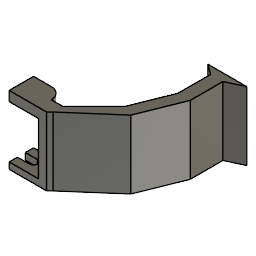
leg sprint 5 (Autodesk Fusion 360 design; units mm, degrees)
Autodesk Fusion 360 part; units mm, degrees
note: some values were not read from the file. Chosen so that the rebuilt part matches the saved one: which face or edge a step refers to; which pieces of a blend or face edit are solid.
sketch "Sketch1" plane through (0, 0, 0) normal (0, 0, 1) x (1, 0, 0)
  line L0 (0, 0) -> (50, 0)
  line L1 (50, 0) -> (50, 15)
  line L2 (50, 15) -> (0, 15)
  line L3 (0, 15) -> (0, 0)
  constraint horizontal L0
  constraint vertical L1
  constraint horizontal L2
  constraint vertical L3
  constraint coincident L0.start L3.end
extrude "Extrude1" add sketch "Sketch1" along normal blind 40 contours L0 L1 L2 L3 picked at (16.666667, 5)
sketch "Sketch2" plane through (0, 0, 0) normal (-1, 0, 0) x (0, -1, 0)
  line L0 (-15, 0) -> (0, 0)
  line L1 (0, 0) -> (0, 40)
  line L2 (0, 40) -> (-15, 40)
  line L3 (-15, 40) -> (-15, 0)
  line L4 (2.957876, 2) -> (-22.207484, 2)
  line L5 (-22.207484, 2) -> (-22.207484, 38.000001)
  line L6 (-22.207484, 38.000001) -> (2.957876, 38.000001)
  line L7 (2.957876, 38.000001) -> (2.957876, 2)
  constraint horizontal L4
  constraint vertical L5
  constraint horizontal L6
  constraint vertical L7
extrude "Extrude2" cut sketch "Sketch2" against normal blind 46 contours L1 L3 L4 L6 picked at (-10, 26)
sketch "Sketch3" plane through (0, 0, 40) normal (0, 0, 1) x (-1, 0, 0)
  line L0 (0, -15) -> (0, 0)
  line L1 (0, 0) -> (-50, 0)
  line L2 (-50, 0) -> (-50, -15)
  line L3 (-50, -15) -> (0, -15)
  circle A0 centre (-7.5, -7.5) radius 2.4
  dimension "d5" = 4.8
  measures "d5" diameter of A0
extrude "Extrude3" cut sketch "Sketch3" against normal blind 50 contours A0 picked at (-7.452057, -6.860244)
sketch "Sketch4" plane through (0, 0, 0) normal (0, 0, -1) x (1, 0, 0)
  circle A0 centre (7.5, -7.5) radius 2.4
  line L0 (0, 0) -> (0, -15)
  line L1 (0, -15) -> (50, -15)
  line L2 (50, -15) -> (50, 0)
  line L3 (50, 0) -> (0, 0)
  circle A1 centre (7.5, -7.5) radius 4
  dimension "d8" = 8
  constraint concentric A0 A1
  measures "d8" diameter of A1
extrude "Extrude4" cut sketch "Sketch4" against normal blind 7 contours A1 picked at (10.951775, -7.698723)
extrude "Extrude5" add 1 faces at (46, 10, 26) along direction (-1, 0, 0) blind 30
extrude "Extrude6" cut 1 faces at (50, 5, 26.666667) along direction (-1, 0, 0) blind 25
chamfer "Chamfer1" distance 7 angle 45 1 edges at (25, 15, 20)
chamfer "Chamfer2" distance 2 angle 45 1 edges at (25, 0, 20)
extrude "Extrude7" add 1 faces at (22.666667, 10.333333, 13.333333) along direction (0.70710678, 0.70710678, 0) blind 30
chamfer "Chamfer3" distance 7 angle 45 1 edges at (39.213203, 36.213203, 20)
extrude "Extrude8" add 1 faces at (40.863119, 31.263456, 13.333333) along direction (0, 1, 0) blind 25
sketch "Sketch5" plane through (0, 0, 0) normal (0, 0, -1) x (1, 0, 0)
  circle A0 centre (7.5, -7.5) radius 4
  line L0 (44.162951, -31.263456) -> (46.213203, -29.213203)
  line L1 (46.213203, -29.213203) -> (25, -8)
  line L2 (25, -8) -> (25, -2)
  line L3 (25, -2) -> (23, 0)
  line L4 (23, 0) -> (0, 0)
  line L5 (0, 0) -> (0, -15)
  line L6 (0, -15) -> (18, -15)
  line L7 (18, -15) -> (34.263456, -31.263456)
  line L8 (34.263456, -31.263456) -> (34.263456, -56.263456)
  line L9 (34.263456, -56.263456) -> (44.162951, -56.263456)
  line L10 (44.162951, -56.263456) -> (44.162951, -31.263456)
  line L11 (44.162951, -31.263456) -> (44.162951, -27.162951)
  line L12 (44.162951, -27.162951) -> (46.213203, -29.213203)
  line L13 (44.162951, -31.263456) -> (46.213203, -29.213203)
  constraint parallel L10 L11
extrude "Extrude9" cut sketch "Sketch5" against normal blind 43 contours L0 L1 L11 L12 L13 picked at (44.846368, -29.213203)
chamfer "Chamfer4" distance 3 angle 45 1 edges at (44.162951, 56.263456, 20)
sketch "Sketch6" plane through (0, 0, 0) normal (0, 0, -1) x (1, 0, 0)
  line L0 (41.162951, -56.263456) -> (44.162951, -53.263456)
  line L1 (44.162951, -53.263456) -> (44.162951, -27.162951)
  line L2 (44.162951, -27.162951) -> (25, -8)
  line L3 (25, -8) -> (25, -2)
  line L4 (25, -2) -> (23, 0)
  line L5 (23, 0) -> (0, 0)
  line L6 (0, 0) -> (0, -15)
  line L7 (0, -15) -> (18, -15)
  line L8 (18, -15) -> (34.263456, -31.263456)
  line L9 (34.263456, -31.263456) -> (34.263456, -56.263456)
  line L10 (34.263456, -56.263456) -> (41.162951, -56.263456)
  circle A0 centre (7.5, -7.5) radius 4
  circle A1 centre (7.5, -7.5) radius 2.4
  dimension "d25" = 4.8
  constraint concentric A0 A1
  measures "d25" diameter of A1
extrude "Extrude10" add sketch "Sketch6" against normal blind 2 contours A0 picked at (10.951775, -7.698723)
sketch "Sketch7" plane through (0, 0, 38.000001) normal (0, 0, -1) x (1, 0, 0)
  line L0 (16, -15) -> (16, 0)
  line L1 (16, 0) -> (0, 0)
  line L2 (0, 0) -> (0, -15)
  line L3 (0, -15) -> (16, -15)
  circle A0 centre (7.5, -7.5) radius 2.4
  circle A1 centre (7.5, -7.5) radius 4
  dimension "d28" = 8
  constraint concentric A0 A1
  measures "d28" diameter of A1
extrude "Extrude11" cut sketch "Sketch7" against normal blind 3 contours A1 picked at (10.951775, -7.698723)
sketch "Sketch8" plane through (0, 0, 38.000001) normal (0, 0, -1) x (1, 0, 0)
  circle A0 centre (7.5, -7.5) radius 4
  line L0 (16, -15) -> (16, 0)
  line L1 (16, 0) -> (0, 0)
  line L2 (0, 0) -> (0, -15)
  line L3 (0, -15) -> (16, -15)
  circle A1 centre (7.5, -7.5) radius 4
  constraint concentric A0 A1
extrude "Extrude12" add sketch "Sketch8" along normal blind 2 and the other way blind 2 contours A0 A1 picked at (6.101654, -8.048811)
extrude "Extrude13" cut 1 faces at (36.563288, 56.263456, 26.666667) along direction (0, -1, 0) blind 25
sketch "Sketch9" plane through (0, 0, 40) normal (0, 0, 1) x (-1, 0, 0)
  line L0 (-41.162951, -56.263456) -> (-41.162951, -31.263456)
  line L1 (-41.162951, -31.263456) -> (-34.263456, -31.263456)
  line L2 (-34.263456, -31.263456) -> (-18, -15)
  line L3 (-18, -15) -> (0, -15)
  line L4 (0, -15) -> (0, 0)
  line L5 (0, 0) -> (-23, 0)
  line L6 (-23, 0) -> (-25, -2)
  line L7 (-25, -2) -> (-25, -8)
  line L8 (-25, -8) -> (-44.162951, -27.162951)
  line L9 (-44.162951, -27.162951) -> (-44.162951, -53.263456)
  line L10 (-44.162951, -53.263456) -> (-41.162951, -56.263456)
extrude "Extrude14" cut 1 faces at (41.162951, 47.930123, 13.333333) along direction (1, 0, 0) blind 26
sketch "Sketch10" plane through (0, 0, 40) normal (0, 0, 1) x (-1, 0, 0)
  line L0 (-44.000001, -27) -> (-34.000001, -31)
  line L1 (-34.000001, -31) -> (-34.243008, -31.24155)
  line L2 (-34.243008, -31.24155) -> (-44.199999, -31.24155)
  line L3 (-44.199999, -31.24155) -> (-44.199999, -27.099999)
  line L4 (-44.199999, -27.099999) -> (-44.000001, -27)
  constraint horizontal L2
  constraint perpendicular L2 L3
extrude "Extrude15" cut sketch "Sketch10" against normal blind 45 contours L0 L1 L2 L3 L4 picked at (-40.814336, -29.8277)
delete_face "DeleteFace1" 1 faces at (40.863119, 31.263456, 13.333333)
delete_face "DeleteFace2" 1 faces at (40.856303, 34.548684, 40)
extrude "Extrude16" add 2 faces at (40.666667, 28.333334, 36.161338) (40.666667, 28.333334, 18.989342) along direction (0.37139068, 0.92847669, 0) blind 40
chamfer "Chamfer5" distance 5 angle 45 1 edges at (58.855628, 64.139068, 20)
extrude "Extrude17" add 1 faces at (13.966667, 7.5, 2) along direction (0, 0, 1) blind 4
extrude "Extrude18" cut 1 faces at (46.618101, 52.878584, 0) along direction (0, 0, 1) blind 2
extrude "Extrude19" cut 1 faces at (16, 10, 16.666667) along direction (1, 0, 0) blind 2
sketch "Sketch11" plane through (0, 0, 40) normal (0, 0, 1) x (-1, 0, 0)
  line L0 (-56.998674, -59.496685) -> (-54.213244, -65.996021)
  line L1 (-54.213244, -65.996021) -> (-48.855628, -68.139068)
  line L2 (-48.855628, -68.139068) -> (-34.000001, -31)
  line L3 (-34.000001, -31) -> (-18, -15)
  line L4 (-18, -15) -> (0, -15)
  line L5 (0, -15) -> (0, 0)
  line L6 (0, 0) -> (-23, 0)
  line L7 (-23, 0) -> (-25, -2)
  line L8 (-25, -2) -> (-25, -8)
  line L9 (-25, -8) -> (-44.000001, -27)
  line L10 (-44.000001, -27) -> (-56.998674, -59.496685)
  line L11 (-56.998674, -59.496685) -> (-60.937867, -50.305234)
  line L12 (-60.937867, -50.305234) -> (-50.499337, -24.208909)
  line L13 (-50.499337, -24.208909) -> (-25, -2)
  line L14 (-18, -15) -> (-18, -8)
  line L15 (-18, -8) -> (-25, -8)
  dimension "d50" = 10
  constraint parallel L0 L11
  constraint parallel L10 L12
  constraint coincident L7.end L8.start
  constraint coincident L3.end L4.start
  constraint perpendicular L4 L14
  constraint coincident L8.end L9.start
extrude "Extrude20" add sketch "Sketch11" against normal blind 38 contours L8 L9 L10 L11 L12 L13 picked at (-53.978847, -45.60064)
extrude "Extrude21" cut sketch "Sketch11" against normal blind 40 contours L0 L1 L2 L3 L9 L10 L14 L15 picked at (-46.618101, -52.878584)
extrude "Extrude22" add sketch "Sketch11" along normal blind 2 contours L8 L9 L10 L11 L12 L13 | L4 L5 L6 L7 L8 L14 L15 picked at (-53.978847, -45.60064) picked at (-6, -7.666667)
fillet "Fillet1" radius 7 2 edges at (18, 15, 4) (18, 15, 40)
sketch "Sketch15" plane through (0, 0, 42) normal (0, 0, 1) x (-1, 0, 0)
  arc A0 (-18, -8) -> (-11, -15) centre (-11, -8) ccw
  line L0 (-11, -15) -> (0, -15)
  line L1 (0, -15) -> (0, 0)
  line L2 (0, 0) -> (-23, 0)
  line L3 (-23, 0) -> (-25, -2)
  line L4 (-25, -2) -> (-50.499337, -24.208909)
  line L5 (-50.499337, -24.208909) -> (-60.937867, -50.305234)
  line L6 (-60.937867, -50.305234) -> (-56.998674, -59.496685)
  line L7 (-56.998674, -59.496685) -> (-44.000001, -27)
  line L8 (-44.000001, -27) -> (-25, -8)
  line L9 (-25, -8) -> (-18, -8)
  line L10 (-60.937867, -50.305234) -> (-53.322094, -50.305234)
  line L11 (-53.322094, -50.305234) -> (-56.998674, -59.496685)
  line L12 (-61.161175, -50.305234) -> (-56.998674, -59.496685)
  line L13 (-61.161175, -50.305234) -> (-60.899999, -50.305234)
  constraint horizontal L10
  constraint parallel L10 L13
extrude "Extrude23" cut sketch "Sketch15" against normal blind 41 contours L6 L7 L10 L11 L13 picked at (-57.073589, -53.369051)
extrude "Extrude24" add 1 faces at (58.399276, 50.305234, 28.666667) along direction (0, 1, 0) blind 20
sketch "Sketch16" plane through (0, 0, 2) normal (0, 0, -1) x (1, 0, 0)
  circle A0 centre (7.5, -7.5) radius 2.4
  line L0 (60.937867, -50.305234) -> (50.499337, -24.208909)
  line L1 (50.499337, -24.208909) -> (25, -2)
  line L2 (25, -2) -> (23, 0)
  line L3 (23, 0) -> (0, 0)
  line L4 (0, 0) -> (0, -15)
  line L5 (0, -15) -> (11, -15)
  arc A1 (11, -15) -> (18, -8) centre (11, -8) ccw
  line L6 (18, -8) -> (25, -8)
  line L7 (25, -8) -> (44.000001, -27)
  line L8 (44.000001, -27) -> (53.322094, -50.305234)
  line L9 (53.322094, -50.305234) -> (53.322094, -70.305234)
  line L10 (53.322094, -70.305234) -> (60.937867, -70.305234)
  line L11 (60.937867, -70.305234) -> (60.937867, -50.305234)
  line L12 (71.000001, -75.000001) -> (60.937867, -70.305234)
  line L13 (53.322094, -70.305234) -> (47.000001, -75.000001)
  line L14 (47.000001, -75.000001) -> (71.000001, -75.000001)
  constraint perpendicular L9 L14
extrude "Extrude25" add sketch "Sketch16" against normal blind 40 contours L10 L12 L13 L14 picked at (59.645956, -73.435079)
extrude "Extrude31" cut 1 faces at (6.101654, 8.048811, 36.000001) along direction (0, 0, 1) blind 1
sketch "Sketch17" plane through (0, 0, 2) normal (0, 0, -1) x (1, 0, 0)
  circle A0 centre (7.5, -7.5) radius 2.4
  line L0 (60.937867, -50.305234) -> (50.499337, -24.208909)
  line L1 (50.499337, -24.208909) -> (25, -2)
  line L2 (25, -2) -> (23, 0)
  line L3 (23, 0) -> (0, 0)
  line L4 (0, 0) -> (0, -15)
  line L5 (0, -15) -> (11, -15)
  arc A1 (11, -15) -> (18, -8) centre (11, -8) ccw
  line L6 (18, -8) -> (25, -8)
  line L7 (25, -8) -> (44.000001, -27)
  line L8 (44.000001, -27) -> (53.322094, -50.305234)
  line L9 (53.322094, -50.305234) -> (53.322094, -70.305234)
  line L10 (53.322094, -70.305234) -> (47.000001, -75.000001)
  line L11 (47.000001, -75.000001) -> (71.000001, -75.000001)
  line L12 (71.000001, -75.000001) -> (60.937867, -70.305234)
  line L13 (60.937867, -70.305234) -> (60.937867, -50.305234)
  line L14 (7.5, -5.1) -> (0, -5.1)
  line L15 (7.5, -9.9) -> (0, -9.9)
  line L16 (0, -9.9) -> (0, -5.1)
  constraint coincident A0 L14.start
  constraint coincident L4 L14.end
  constraint perpendicular L4 L14
  constraint coincident A0 L15.start
  constraint coincident L4 L15.end
  constraint perpendicular L4 L15
extrude "Extrude32" cut sketch "Sketch17" against normal blind 4 contours A0 L4 L14 L15 L16 picked at (1.702237, -7.440216)
sketch "Sketch18" plane through (0, 0, 37.000001) normal (0, 0, -1) x (1, 0, 0)
  circle A0 centre (7.5, -7.5) radius 4
  line L0 (8.5, -7.5) -> (8.5, -3.627017)
  line L1 (8.5, -7.5) -> (8.5, -11.372983)
  line L2 (6.5, -7.5) -> (6.5, -3.627017)
  line L3 (6.5, -7.5) -> (6.5, -11.372983)
  constraint vertical L2
  constraint parallel L2 L3
extrude "Extrude33" cut sketch "Sketch18" against normal blind 1 contours A0 L0 L1 | A0 L2 L3 picked at (10.485726, -7.694579) picked at (4.514274, -7.305421)
fillet "Fillet2" radius 1 4 edges at (8.5, 3.627017, 37.500001) (8.5, 11.372983, 37.500001) (6.5, 3.627017, 37.500001) (6.5, 11.372983, 37.500001)
extrude "Extrude34" add 1 faces at (9.667133, 7.666667, 42) along direction (0, 0, 1) blind 2
sketch "Sketch19" plane through (0, 0, 44) normal (0, 0, 1) x (-1, 0, 0)
  line L0 (-53.322094, -50.305234) -> (-44.000001, -27)
  line L1 (-44.000001, -27) -> (-25, -8)
  line L2 (-25, -8) -> (-18, -8)
  arc A0 (-18, -8) -> (-11, -15) centre (-11, -8) ccw
  line L3 (-11, -15) -> (0, -15)
  line L4 (0, -15) -> (0, 0)
  line L5 (0, 0) -> (-23, 0)
  line L6 (-23, 0) -> (-25, -2)
  line L7 (-25, -2) -> (-50.499337, -24.208909)
  line L8 (-50.499337, -24.208909) -> (-60.937867, -50.305234)
  line L9 (-60.937867, -50.305234) -> (-60.937867, -70.305234)
  line L10 (-60.937867, -70.305234) -> (-71.000001, -75.000001)
  line L11 (-71.000001, -75.000001) -> (-47.000001, -75.000001)
  line L12 (-47.000001, -75.000001) -> (-53.322094, -70.305234)
  line L13 (-53.322094, -70.305234) -> (-53.322094, -50.305234)
  line L14 (-60.000001, -75.000001) -> (-60.000001, -74.000001)
  line L15 (-60.000001, -74.000001) -> (-55.000001, -74.000001)
  line L16 (-55.000001, -74.000001) -> (-54.000001, -74.000001)
  line L17 (-54.000001, -74.000001) -> (-54.000001, -75.000001)
  line L18 (-58.000001, -74.000001) -> (-58.000001, -75.000001)
  line L19 (-56.000001, -74.000001) -> (-56.000001, -75.000001)
  constraint perpendicular L11 L14
  constraint perpendicular L14 L15
  constraint perpendicular L11 L17
  constraint perpendicular L11 L18
  constraint perpendicular L11 L19
extrude "Extrude35" [rolled back] along distance -45 taper angle 0
extrude "Extrude26" [suppressed]
extrude "Extrude27" [suppressed]
extrude "Extrude28" [suppressed]
extrude "Extrude29" [suppressed]
extrude "Extrude30" [suppressed]
